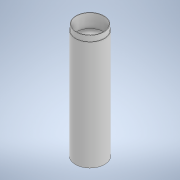
# Autodesk Inventor part: payloadchamber
Saved by Autodesk Inventor 2020.3 (Build 243373000, 373)
## iProperties
Created: 2021-01-23
Part Number: payloadchamber
Material: ABS Plastic
Document SubType Name: Modeling
Designer: 0x6f736f646f
Density: 1.06 g/cm^3
Appearance: Default
Author: 0x6f736f646f
Autodesk Inventor part; units mm, degrees
ref_plane "YZ Plane" through (0, 0, 0) normal (1, 0, 0) x (0, 1, 0)
ref_plane "XY Plane" through (0, 0, 0) normal (0, 0, 1) x (1, 0, 0)
sketch "Sketch1" plane through (0, 0, 0) normal (0, 1, 0) x (-1, 0, 0)
  circle A0 centre (0, 0) radius 25.9
  circle A1 centre (0, 0) radius 25
  circle A2 centre (0, 0) radius 26.8
  circle A3 centre (0, 0) radius 10
  dimension "d0" = 51.8
  dimension "d1" = 50
  dimension "d2" = 53.6
  dimension "d12" = 20
  constraints: 4 centre point, 4 coincident
  measures "d0" diameter of A0
  measures "d1" diameter of A1
  measures "d2" diameter of A2
  measures "d12" diameter of A3
extrude "Extrusion1" add sketch "Sketch1" along normal blind 110 and the other way blind 90 contours A0
extrude "Extrusion2" add sketch "Sketch1" along normal mid plane 200 contours A2
ref_plane "Work Plane1" through (0, 80, 0) normal (0, 1, 0) x (-1, 0, 0)
sketch "Sketch2" plane through (0, 80, 0) normal (0, 1, 0) x (-1, 0, 0)
  circle A0 centre (0, 0) radius 25.9
  circle A1 centre (0, 0) radius 25
  circle A2 centre (0, 0) radius 26.8
  circle A3 centre (0, 0) radius 10
  dimension "d14" = 51.8
  dimension "d15" = 50
  dimension "d16" = 53.6
  dimension "d17" = 20
  constraints: 4 centre point, 4 coincident
  measures "d14" diameter of A0
  measures "d15" diameter of A1
  measures "d16" diameter of A2
  measures "d17" diameter of A3
extrude "Extrusion3" add sketch "Sketch2" along normal blind 5 contours A1 | A3
body "Solid1"
